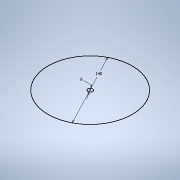
# Autodesk Inventor part: Stepper_Closing_1
Saved by Autodesk Inventor 2022.3 (Build 263350000, 350)
## iProperties
Created: 2023-05-23
Part Number: Stepper_Closing_1
Material: Generic
Document SubType Name: Modeling
Designer: Manuel Hueso Béjar
Density: 1 g/cm^3
Appearance: Default
Author: Manuel Hueso Béjar
Autodesk Inventor part; units mm, degrees
ref_plane "YZ Plane" through (0, 0, 0) normal (1, 0, 0) x (0, 1, 0)
ref_plane "XZ Plane" through (0, 0, 0) normal (0, 1, 0) x (-1, 0, 0)
ref_plane "XY Plane" through (0, 0, 0) normal (0, 0, 1) x (1, 0, 0)
sketch "Sketch1" plane through (0, 0, 0) normal (0, 1, 0) x (-1, 0, 0)
  circle A0 centre (0, 0) radius 32.5
  dimension "d0" = 65
  constraints: 1 centre point, 1 coincident
  measures "d0" diameter of A0
extrude "Extrusion3" add sketch "Sketch1" along normal blind 2
sketch "Sketch3" plane through (0, 2, 0) normal (0, 1, 0) x (1, 0, 0)
  circle A0 centre (0, 0) radius 4
  dimension "d17" = 8
  constraints: 1 centre point, 1 coincident
  measures "d17" diameter of A0
extrude "Extrusion4" add sketch "Sketch3" along normal blind 14
fillet "Fillet2" radius 6 1 edges at (-4, 2, 0)
fillet "Fillet3" radius 2 1 edges at (32.5, 0, 0)
sketch "Sketch4" plane through (0, 0, 0) normal (0, -1, 0) x (1, 0, 0)
  line L0 (32.5, -32.5) -> (-32.5, -32.5) construction
  line L1 (-32.5, -32.5) -> (-32.5, 32.5) construction
  line L2 (-32.5, 32.5) -> (32.5, 32.5) construction
  line L3 (32.5, 32.5) -> (32.5, -32.5) construction
  line L4 (32.5, 32.5) -> (-32.5, 32.5)
  line L5 (-32.5, 32.5) -> (-32.5, -32.5)
  line L6 (-32.5, -32.5) -> (32.5, -32.5)
  line L7 (32.5, -32.5) -> (32.5, 32.5)
  circle A0 centre (0, 0) radius 4 projected
  line L8 (32.5, 32.5) -> (-32.5, -32.5) construction
  line L9 (-32.5, 32.5) -> (32.5, -32.5) construction
  line L10 (12.7634, 15) -> (2.6499, -15)
  line L11 (2.6499, -15) -> (-2.2609, -15)
  line L12 (-2.2609, -15) -> (-12.3744, 15)
  line L13 (-12.3744, 15) -> (-8.1686, 15)
  line L14 (-8.1686, 15) -> (-5.4457, 6.6126)
  line L15 (-5.4457, 6.6126) -> (6.0049, 6.6126)
  line L16 (6.0049, 6.6126) -> (8.7277, 15)
  line L17 (8.7277, 15) -> (12.7634, 15)
  line L18 (-4.3517, 3.2091) -> (0.2917, -10.9157)
  line L19 (0.2917, -10.9157) -> (4.9109, 3.2091)
  line L20 (4.9109, 3.2091) -> (-4.3517, 3.2091)
  dimension "d22" = 65
  dimension "d23" = 65
  dimension "d24" = 65
  dimension "d25" = 65
  dimension "d26" = 0
  dimension "d27" = 0
  constraints: 12 end point, 2 midpoint, 2 parallel, 1 horizontal, 1 perpendicular, 2 other
  measures "d22" distance of L0.start L0.end
  measures "d23" distance of L0.end L1.end
  measures "d24" distance of L6.end L5.end
  measures "d25" distance of L5.end L4.end
  measures "d26" distance between parallel lines of L6 L0
  measures "d27" distance between parallel lines of L5 L1
emboss "Emboss2" sketch "Sketch4" operation cut depth 1 direction (0, 1, 0) contours A0 L19 | L20 A0 | A0 L18 | L10 L11 L12 L13 L14 L15 L16 L17
body "Solid2"
